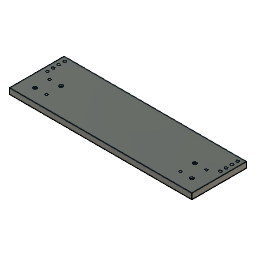
riser top (Autodesk Fusion 360 design; units mm, degrees)
Autodesk Fusion 360 part; units mm, degrees
note: some values were not read from the file. Set by a fixed rule: which face or edge a step refers to.
sketch "Sketch1" plane through (0, 0, 0) normal (0, 0, 1) x (1, 0, 0)
  line L0 (0, 0) -> (320, 0)
  line L1 (320, 0) -> (320, 100)
  line L2 (320, 100) -> (0, 100)
  line L3 (0, 100) -> (0, 0)
  dimension "d1" = 320
  dimension "d2" = 100
  constraint horizontal L0
  constraint vertical L1
  constraint horizontal L2
  constraint vertical L3
  constraint coincident L0.start L3.end
  measures "d1" distance of L0.start L0.end
  measures "d2" distance of L0.start L2.end
extrude "Extrude1" add sketch "Sketch1" along normal blind 10
sketch "Sketch2" plane through (0, 0, 10) normal (0, 0, 1) x (-1, 0, 0)
  line L0 (0, -100) -> (0, 0)
  line L1 (0, 0) -> (-320, 0)
  line L2 (-320, 0) -> (-320, -100)
  line L3 (-320, -100) -> (0, -100)
  circle A0 centre (-11, -90) radius 2.25
  circle A1 centre (-309, -90) radius 2.25
  circle A2 centre (-11, -80) radius 2.25
  circle A3 centre (-309, -80) radius 2.25
  circle A4 centre (-11, -70) radius 2.25
  circle A5 centre (-11, -60) radius 2.075
  circle A6 centre (-309, -70) radius 2.25
  circle A7 centre (-309, -60) radius 2.25
  dimension "d5" = 4.5
  dimension "d6" = 4.5
  dimension "d7" = 298
  dimension "d8" = 11
  dimension "d9" = 10
  dimension "d10" = 4.5
  dimension "d11" = 4.5
  dimension "d13" = 4.5
  dimension "d14" = 4.5
  dimension "d16" = 4.15
  dimension "d17" = 4.5
  measures "d5" diameter of A0
  measures "d6" diameter of A1
  measures "d7" distance of A0.centre A1.centre
  measures "d8" distance of L0 A0.centre
  measures "d9" distance of L3 A0.centre
  measures "d10" diameter of A2
  measures "d11" diameter of A3
  measures "d13" diameter of A4
  measures "d14" diameter of A6
  measures "d16" diameter of A5
  measures "d17" diameter of A7
extrude "Extrude2" cut sketch "Sketch2" against normal blind 30 contours A0 | A1 | A2 | A3 | A4 | A5 | A6 | A7
sketch "Sketch4" plane through (0, 0, 10) normal (0, 0, 1) x (-1, 0, 0)
  line L0 (0, -100) -> (0, 0)
  line L1 (0, 0) -> (-320, 0)
  line L2 (-320, 0) -> (-320, -100)
  line L3 (-320, -100) -> (0, -100)
  line L4 (-317, -3) -> (-3, -3)
  line L5 (-3, -3) -> (-3, -97)
  line L6 (-3, -97) -> (-317, -97)
  line L7 (-317, -97) -> (-317, -3)
  circle A0 centre (-309, -80) radius 2.25
  circle A1 centre (-11, -80) radius 2.25
  circle A2 centre (-11, -70) radius 2.25
  circle A3 centre (-309, -70) radius 2.25
  circle A4 centre (-309, -90) radius 2.25
  circle A5 centre (-11, -90) radius 2.25
  circle A6 centre (-11, -60) radius 2.075
  circle A7 centre (-309, -60) radius 2.25
  constraint horizontal L4
  constraint vertical L5
  constraint horizontal L6
  constraint vertical L7
extrude "Extrude4" add sketch "Sketch4" along normal blind 5 contours L0 L1 L2 L3
sketch "Sketch5" plane through (0, 0, 10) normal (0, 0, 1) x (-1, 0, 0)
  line L0 (-3, -97) -> (-3, -3)
  line L1 (-3, -3) -> (-317, -3)
  line L2 (-317, -3) -> (-317, -97)
  line L3 (-317, -97) -> (-3, -97)
  circle A0 centre (-25, -50) radius 2.075
  circle A1 centre (-25, -25) radius 2.075
  circle A2 centre (-295, -50) radius 2.075
  circle A3 centre (-295, -25) radius 2.075
  circle A4 centre (-309, -80) radius 2.25
  circle A5 centre (-11, -80) radius 2.25
  circle A6 centre (-11, -70) radius 2.25
  circle A7 centre (-309, -70) radius 2.25
  circle A8 centre (-309, -90) radius 2.25
  circle A9 centre (-11, -90) radius 2.25
  circle A10 centre (-11, -60) radius 2.075
  circle A11 centre (-309, -60) radius 2.25
  dimension "d32" = 4.15
  dimension "d33" = 4.15
  dimension "d34" = 4.15
  dimension "d35" = 4.15
  measures "d32" diameter of A0
  measures "d33" diameter of A1
  measures "d34" diameter of A2
  measures "d35" diameter of A3
extrude "Extrude5" add sketch "Sketch5" along normal blind 3 contours A0 | A1 | A2 | A3
sketch "Sketch6" plane through (0, 0, 10) normal (0, 0, 1) x (-1, 0, 0)
  circle A0 centre (-295, -25) radius 2.075
  circle A1 centre (-25, -50) radius 2.075
  circle A2 centre (-295, -50) radius 2.075
  circle A3 centre (-25, -25) radius 2.075
  line L0 (-3, -97) -> (-3, -3)
  line L1 (-3, -3) -> (-317, -3)
  line L2 (-317, -3) -> (-317, -97)
  line L3 (-317, -97) -> (-3, -97)
  circle A4 centre (-45, -50) radius 2.075
  circle A5 centre (-45, -25) radius 2.075
  circle A6 centre (-275, -50) radius 2.075
  circle A7 centre (-275, -25) radius 2.075
  circle A8 centre (-309, -80) radius 2.25
  circle A9 centre (-11, -80) radius 2.25
  circle A10 centre (-11, -70) radius 2.25
  circle A11 centre (-309, -70) radius 2.25
  circle A12 centre (-309, -90) radius 2.25
  circle A13 centre (-11, -90) radius 2.25
  circle A14 centre (-11, -60) radius 2.075
  circle A15 centre (-309, -60) radius 2.25
  dimension "d38" = 4.15
  dimension "d39" = 4.15
  dimension "d40" = 4.15
  dimension "d41" = 4.15
  measures "d38" diameter of A4
  measures "d39" diameter of A5
  measures "d40" diameter of A6
  measures "d41" diameter of A7
extrude "Extrude6" cut sketch "Sketch6" against normal blind 3 contours A4 | A5 | A6 | A7
extrude "Extrude7" cut 1 faces at (212.3333, 1, 15) along direction (0, 0, -1) blind 15
extrude "Extrude8" cut 4 faces at (24.3391, 50.0023, 13) (25.1539, 24.4763, 13) (295.5715, 25.5958, 13) (294.4285, 49.4042, 13) along direction (0, 0, -1) blind 6
extrude "Extrude9" cut 8 faces at (24.3391, 50.0023, 7) (44.8839, 51.5498, 7) (44.3461, 25.504, 7) (25.1539, 24.4763, 7) (275.5715, 50.5958, 7) (274.4285, 24.4042, 7) (295.5715, 25.5958, 7) (294.4285, 49.4042, 7) along direction (0, 0, -1) blind 10
sketch "Sketch8" plane through (0, 0, 10) normal (0, 0, 1) x (-1, 0, 0)
  circle A0 centre (-45, -25) radius 2.075
  circle A1 centre (-275, -50) radius 2.075
  circle A2 centre (-45, -50) radius 2.075
  circle A3 centre (-275, -25) radius 2.075
  circle A4 centre (-295, -25) radius 2.075
  circle A5 centre (-25, -50) radius 2.075
  circle A6 centre (-295, -50) radius 2.075
  circle A7 centre (-25, -25) radius 2.075
  line L0 (-3, -97) -> (-3, -3)
  line L1 (-3, -3) -> (-317, -3)
  line L2 (-317, -3) -> (-317, -97)
  line L3 (-317, -97) -> (-3, -97)
  circle A8 centre (-309, -80) radius 2.25
  circle A9 centre (-11, -80) radius 2.25
  circle A10 centre (-11, -70) radius 2.25
  circle A11 centre (-309, -70) radius 2.25
  circle A12 centre (-309, -90) radius 2.25
  circle A13 centre (-11, -90) radius 2.25
  circle A14 centre (-11, -60) radius 2.075
  circle A15 centre (-309, -60) radius 2.25
  circle A16 centre (-25, -50) radius 3
  circle A17 centre (-45, -50) radius 3
  circle A18 centre (-25, -25) radius 3
  circle A19 centre (-45, -25) radius 3
  circle A20 centre (-275, -50) radius 3
  circle A21 centre (-295, -50) radius 3
  circle A22 centre (-275, -25) radius 3
  circle A23 centre (-295, -25) radius 3
  dimension "d52" = 6
  dimension "d53" = 6
  dimension "d54" = 6
  dimension "d55" = 6
  dimension "d56" = 6
  dimension "d57" = 6
  constraint concentric A5 A16
  constraint concentric A7 A18
  constraint concentric A0 A19
  constraint concentric A1 A20
  constraint concentric A6 A21
  constraint concentric A3 A22
  constraint concentric A4 A23
  measures "d52" diameter of A17
  measures "d53" diameter of A19
  measures "d54" diameter of A20
  measures "d55" diameter of A21
  measures "d56" diameter of A22
  measures "d57" diameter of A23
extrude "Extrude10" cut sketch "Sketch8" against normal blind 2 contours A16 | A17 | A18 | A19 | A20 | A21 | A22 | A23
sketch "Sketch10" plane through (0, 0, 0) normal (0, 0, -1) x (1, 0, 0)
  circle A0 centre (295, -25) radius 2.075
  circle A1 centre (275, -50) radius 2.075
  circle A2 centre (45, -25) radius 2.075
  circle A3 centre (25, -50) radius 2.075
  circle A4 centre (45, -50) radius 2.075
  circle A5 centre (25, -25) radius 2.075
  circle A6 centre (275, -25) radius 2.075
  circle A7 centre (295, -50) radius 2.075
  line L0 (317, -97) -> (317, -3)
  line L1 (317, -3) -> (3, -3)
  line L2 (3, -3) -> (3, -97)
  line L3 (3, -97) -> (317, -97)
  circle A8 centre (309, -80) radius 2.25
  circle A9 centre (11, -80) radius 2.25
  circle A10 centre (11, -70) radius 2.25
  circle A11 centre (309, -70) radius 2.25
  circle A12 centre (309, -90) radius 2.25
  circle A13 centre (11, -90) radius 2.25
  circle A14 centre (11, -60) radius 2.075
  circle A15 centre (309, -60) radius 2.25
  circle A16 centre (45, -25) radius 3
  circle A17 centre (25, -50) radius 3
  circle A18 centre (275, -25) radius 3
  circle A19 centre (295, -50) radius 3
  constraint concentric A2 A16
  constraint concentric A3 A17
  constraint concentric A6 A18
  constraint concentric A7 A19
extrude "Extrude11" add 4 faces at (297.1308, 48.3669, 8) (274.2582, 22.4199, 8) (42.3272, 25.2521, 8) (22.3272, 50.2521, 8) along direction (0, 0, 1) blind 2
sketch "Sketch11" plane through (0, 0, 10) normal (0, 0, 1) x (-1, 0, 0)
  circle A0 centre (-25, -50) radius 2.075
  circle A1 centre (-275, -25) radius 2.075
  circle A2 centre (-295, -50) radius 2.075
  circle A3 centre (-45, -25) radius 2.075
  circle A4 centre (-45, -50) radius 3
  circle A5 centre (-25, -25) radius 3
  circle A6 centre (-275, -50) radius 3
  circle A7 centre (-295, -25) radius 3
  line L0 (-3, -97) -> (-3, -3)
  line L1 (-3, -3) -> (-317, -3)
  line L2 (-317, -3) -> (-317, -97)
  line L3 (-317, -97) -> (-3, -97)
  circle A8 centre (-309, -80) radius 2.25
  circle A9 centre (-11, -80) radius 2.25
  circle A10 centre (-11, -70) radius 2.25
  circle A11 centre (-309, -70) radius 2.25
  circle A12 centre (-309, -90) radius 2.25
  circle A13 centre (-11, -90) radius 2.25
  circle A14 centre (-11, -60) radius 2.075
  circle A15 centre (-309, -60) radius 2.25
extrude "Extrude12" cut sketch "Sketch10" against normal blind 2 contours A16 | A17 | A18 | A19
